Autodesk Inventor part; units mm, degrees
(part 2 of 2)
  circle A153 centre (-78.9982, -45.7929) radius 8 projected
  line L91 (-61.2813, 11.0455) -> (-50.1121, 17.3163) projected
  arc A154 (-102.4384, -34.1927) -> (-61.2813, 11.0455) centre (-111.1209, 15.0476) ccw projected
  line L92 (-102.4384, -34.1927) -> (-110.7406, -35.6566) projected
  line L93 (-110.7406, -35.6566) -> (-106.6609, -58.794) projected
  line L94 (-106.6609, -58.794) -> (-103.0049, -58.1494) projected
  arc A155 (-103.0049, -58.1494) -> (-82.3987, -72.578) centre (-78.9982, -45.7929) ccw projected
  line L95 (-82.3987, -72.578) -> (-81.7541, -76.234) projected
  line L96 (-81.7541, -76.234) -> (-73.8756, -74.8448) projected
  line L97 (-73.8756, -74.8448) -> (-28.2963, -90.7089) projected
  line L98 (-28.2963, -90.7089) -> (-30.7152, -97.3549) projected
  line L99 (-30.7152, -97.3549) -> (-15.0425, -100.6253) projected
  arc A156 (-15.0425, -100.6253) -> (-9.8606, -100.8097) centre (-10.3402, -41.375) ccw projected
  line L100 (-9.8606, -100.8097) -> (-9.8684, -99.8389) projected
  arc A157 (-7.953, -97.8245) -> (-9.8684, -99.8389) centre (-7.8685, -99.8228) ccw projected
  arc A158 (-7.953, -97.8245) -> (0.7138, -96.7831) centre (-10.3402, -41.375) ccw projected
  arc A159 (3.052, -98.2863) -> (0.7138, -96.7831) centre (1.1051, -98.7445) ccw projected
  line L101 (3.052, -98.2863) -> (3.358, -99.5868) projected
  arc A160 (3.358, -99.5868) -> (9.3677, -97.836) centre (-10.3402, -41.375) ccw projected
  line L102 (9.3677, -97.836) -> (20.2434, -92.7646) projected
  arc A161 (20.2434, -92.7646) -> (25.4476, -89.2862) centre (-10.3402, -41.375) ccw projected
  line L103 (25.4476, -89.2862) -> (24.6481, -88.2159) projected
  arc A162 (24.9994, -85.4585) -> (24.6481, -88.2159) centre (26.2504, -87.019) ccw projected
  arc A163 (24.9994, -85.4585) -> (31.3681, -79.4888) centre (-10.3402, -41.375) ccw projected
  arc A164 (34.1424, -79.3163) -> (31.3681, -79.4888) centre (32.8445, -80.838) ccw projected
  line L104 (34.1424, -79.3163) -> (34.8811, -79.9463) projected
  arc A165 (34.8811, -79.9463) -> (38.0707, -75.8583) centre (-10.3402, -41.375) ccw projected
  line L105 (38.0707, -75.8583) -> (45.6397, -61.75) projected
  line L106 (45.6397, -61.75) -> (38.9936, -59.3311) projected
  arc A166 (38.9936, -59.3311) -> (35.1261, -15.125) centre (-10.3402, -41.375) ccw projected
  line L107 (35.1261, -15.125) -> (41.2511, -11.5887) projected
  line L108 (41.2511, -11.5887) -> (31.3473, 0.9908) projected
  arc A167 (31.3473, 0.9908) -> (27.4962, 4.4629) centre (-10.3402, -41.375) ccw projected
  line L109 (27.4962, 4.4629) -> (26.8782, 3.7142) projected
  arc A168 (24.1161, 3.4024) -> (26.8782, 3.7142) centre (25.3358, 4.9874) ccw projected
  arc A169 (24.1161, 3.4024) -> (16.8075, 8.1755) centre (-10.3402, -41.375) ccw projected
  arc A170 (15.9827, 10.8299) -> (16.8075, 8.1755) centre (17.7685, 9.9295) ccw projected
  line L110 (15.9827, 10.8299) -> (16.5842, 12.0228) projected
  arc A171 (16.5842, 12.0228) -> (10.8551, 14.5447) centre (-10.3402, -41.375) ccw projected
  line L111 (10.8551, 14.5447) -> (-0.736, 17.6505) projected
  arc A172 (-0.736, 17.6505) -> (-6.9585, 18.3311) centre (-10.3402, -41.375) ccw projected
  line L112 (-6.9585, 18.3311) -> (-7.034, 16.9972) projected
  arc A173 (-9.0756, 15.1108) -> (-7.034, 16.9972) centre (-9.0308, 17.1103) ccw projected
  arc A174 (-9.0756, 15.1108) -> (-17.7916, 14.6315) centre (-10.3402, -41.375) ccw projected
  arc A175 (-20.0277, 16.2826) -> (-17.7916, 14.6315) centre (-18.0553, 16.614) ccw projected
  line L113 (-20.0277, 16.2826) -> (-20.1886, 17.24) projected
  arc A176 (-20.1886, 17.24) -> (-25.2597, 16.1586) centre (-10.3402, -41.375) ccw projected
  line L114 (-25.2597, 16.1586) -> (-40.1265, 10.2163) projected
  line L115 (-40.1265, 10.2163) -> (-50.1121, 17.3163) projected
  circle A177 centre (-103.9086, -54.247) radius 1.5 projected
  circle A178 centre (-13.7974, -97.2048) radius 1.5 projected
  circle A179 centre (20.8436, -88.2521) radius 1.5 projected
  circle A180 centre (28.1949, -0.8291) radius 1.5 projected
  circle A181 centre (-4.0964, 14.5795) radius 1.5 projected
  circle A182 centre (-23.4396, 13.0063) radius 1.5 projected
  circle A183 centre (12.2297, 10.2049) radius 1.5 projected
  circle A184 centre (34.6501, -74.6133) radius 1.5 projected
  circle A185 centre (5.5251, -95.3952) radius 1.5 projected
  circle A186 centre (-78.4226, -72.0925) radius 1.5 projected
  circle A187 centre (-10.3402, -41.375) radius 32.5 projected
  circle A188 centre (-78.9982, -45.7929) radius 12.5
  circle A189 centre (-78.9982, -45.7929) radius 21
  line L116 (-78.9982, -45.7929) -> (-99.6792, -49.4396)
  line L117 (-78.9982, -45.7929) -> (-86.1806, -65.5265)
  point P0 (0, 0)
  point P1 (-83.2735, -57.5391)
  point P2 (-91.3083, -47.9635)
  dimension "d58" = 25
  dimension "d59" = 42
  dimension "d60" = 60
  constraints: 4 end point, 2 centre point, 2 coincident, 2 point on circle, 1 parallel
  measures "d58" diameter of A188
  measures "d59" diameter of A189
  measures "d60" angle of L116 L117
extrude "Extrusion10" cut sketch "Sketch12" against normal blind 5 contours L116 A188 L117 A189
thicken "Thicken1" operation add thickness 1 both sides no extend neighbours yes toward (-0.6427876, -0.7660444, 0) faces at (-87.0331, -55.3685, 1.6667)
sketch "Sketch13" plane through (0, 0, 5) normal (0, 0, 1) x (1, 0, 0)
  line L0 (-83.6155, -58.4788) -> (-86.1806, -65.5265) projected
  arc A0 (-99.6792, -49.4396) -> (-86.1806, -65.5265) centre (-78.9982, -45.7929) ccw projected
  line L1 (-99.6792, -49.4396) -> (-92.2931, -48.1372) projected
  arc A1 (-92.2931, -48.1372) -> (-83.6155, -58.4788) centre (-78.9982, -45.7929) ccw projected
  arc A2 (-21.8035, -78.1288) -> (-9.3616, -79.8626) centre (-10.3402, -41.375) ccw projected
  line L2 (-9.3616, -79.8626) -> (-9.1582, -87.86) projected
  arc A3 (-24.6798, -85.6088) -> (-9.1582, -87.86) centre (-10.3402, -41.375) ccw projected
  line L3 (-24.6798, -85.6088) -> (-21.8314, -78.2051) projected
  arc A4 (-21.8314, -78.2051) -> (-21.8035, -78.1288) centre (-24.1646, -77.3074) ccw projected
  arc A5 (1.123, -4.6212) -> (-11.3188, -2.8874) centre (-10.3402, -41.375) ccw projected
  line L4 (-11.3188, -2.8874) -> (-11.6366, 9.6085) projected
  arc A6 (5.6174, 7.0642) -> (-11.6366, 9.6085) centre (-10.3402, -41.375) ccw projected
  line L5 (5.6174, 7.0642) -> (1.1509, -4.5449) projected
  arc A7 (1.1509, -4.5449) -> (1.123, -4.6212) centre (3.4842, -5.4426) ccw projected
  arc A8 (4.1075, -90.2858) -> (19.7424, -82.5579) centre (-10.3402, -41.375) ccw projected
  line L6 (4.1075, -90.2858) -> (0.5664, -78.2978) projected
  arc A9 (0.5664, -78.2978) -> (11.8719, -72.8214) centre (-10.3402, -41.375) ccw projected
  arc A10 (11.8719, -72.8214) -> (11.9219, -72.8853) centre (13.8659, -71.3135) ccw projected
  line L7 (11.9219, -72.8853) -> (19.7424, -82.5579) projected
  arc A11 (-59.922, -29.4317) -> (-61.047, -46.8359) centre (-10.3402, -41.375) ccw projected
  line L8 (-59.922, -29.4317) -> (-47.7696, -32.359) projected
  arc A12 (-47.7696, -32.359) -> (-48.6796, -44.888) centre (-10.3402, -41.375) ccw projected
  arc A13 (-48.6796, -44.888) -> (-48.76, -44.8994) centre (-48.3708, -47.3689) ccw projected
  line L9 (-48.76, -44.8994) -> (-61.047, -46.8359) projected
  arc A14 (-36.4384, -13.0706) -> (-44.1607, -22.9787) centre (-10.3402, -41.375) ccw projected
  line L10 (-44.1607, -22.9787) -> (-55.1414, -17.0059) projected
  arc A15 (-44.311, -3.3357) -> (-55.1414, -17.0059) centre (-10.3402, -41.375) ccw projected
  line L11 (-44.311, -3.3357) -> (-36.4904, -13.0083) projected
  arc A16 (-36.4904, -13.0083) -> (-36.4384, -13.0706) centre (-34.5464, -11.4365) ccw projected
  arc A17 (34.8667, -52.2645) -> (35.9156, -36.6156) centre (-10.3402, -41.375) ccw projected
  line L12 (34.8667, -52.2645) -> (27.0892, -50.391) projected
  arc A18 (27.0892, -50.391) -> (27.9992, -37.862) centre (-10.3402, -41.375) ccw projected
  arc A19 (27.9992, -37.862) -> (28.0796, -37.8506) centre (27.6903, -35.3811) ccw projected
  line L13 (28.0796, -37.8506) -> (35.9156, -36.6156) projected
  arc A20 (-26.4675, -76.3344) -> (-26.4979, -76.4097) centre (-24.1646, -77.3074) ccw projected
  line L14 (-26.4979, -76.4097) -> (-29.3464, -83.8134) projected
  arc A21 (-42.3743, -75.0806) -> (-29.3464, -83.8134) centre (-10.3402, -41.375) ccw projected
  line L15 (-42.3743, -75.0806) -> (-36.863, -69.2818) projected
  arc A22 (-36.863, -69.2818) -> (-26.4675, -76.3344) centre (-10.3402, -41.375) ccw projected
  arc A23 (5.7871, -6.4156) -> (5.8175, -6.3403) centre (3.4842, -5.4426) ccw projected
  line L16 (5.8175, -6.3403) -> (10.2839, 5.2688) projected
  arc A24 (24.7939, -4.4075) -> (10.2839, 5.2688) centre (-10.3402, -41.375) ccw projected
  line L17 (24.7939, -4.4075) -> (16.1826, -13.4682) projected
  arc A25 (16.1826, -13.4682) -> (5.7871, -6.4156) centre (-10.3402, -41.375) ccw projected
  line L18 (23.6306, -79.4143) -> (15.81, -69.7417) projected
  arc A26 (15.81, -69.7417) -> (15.7579, -69.6794) centre (13.8659, -71.3135) ccw projected
  arc A27 (15.7579, -69.6794) -> (23.4803, -59.7713) centre (-10.3402, -41.375) ccw projected
  line L19 (23.4803, -59.7713) -> (34.461, -65.7441) projected
  arc A28 (23.6306, -79.4143) -> (34.461, -65.7441) centre (-10.3402, -41.375) ccw projected
  line L20 (-60.2686, -51.7749) -> (-47.9816, -49.8384) projected
  arc A29 (-47.9816, -49.8384) -> (-47.9016, -49.8245) centre (-48.3708, -47.3689) ccw projected
  arc A30 (-47.9016, -49.8245) -> (-43.1821, -61.4663) centre (-10.3402, -41.375) ccw projected
  line L21 (-43.1821, -61.4663) -> (-53.8451, -67.9894) projected
  arc A31 (-60.2686, -51.7749) -> (-53.8451, -67.9894) centre (-10.3402, -41.375) ccw projected
  arc A32 (-32.5523, -9.9286) -> (-32.6023, -9.8647) centre (-34.5464, -11.4365) ccw projected
  line L22 (-32.6023, -9.8647) -> (-40.4229, -0.1921) projected
  arc A33 (-24.7879, 7.5358) -> (-40.4229, -0.1921) centre (-10.3402, -41.375) ccw projected
  line L23 (-24.7879, 7.5358) -> (-21.2468, -4.4522) projected
  arc A34 (-21.2468, -4.4522) -> (-32.5523, -9.9286) centre (-10.3402, -41.375) ccw projected
  line L24 (35.1371, -31.6766) -> (27.3011, -32.9116) projected
  arc A35 (27.3011, -32.9116) -> (27.2212, -32.9255) centre (27.6903, -35.3811) ccw projected
  arc A36 (27.2212, -32.9255) -> (22.5017, -21.2837) centre (-10.3402, -41.375) ccw projected
  line L25 (22.5017, -21.2837) -> (29.326, -17.1089) projected
  arc A37 (35.1371, -31.6766) -> (29.326, -17.1089) centre (-10.3402, -41.375) ccw projected
  circle A38 centre (-81.1726, -30.4864) radius 2.1 projected
  circle A39 centre (-65.5868, -14.9006) radius 2.1 projected
  circle A40 centre (-101.657, -38.6244) radius 2.1 projected
  circle A41 centre (-57.4488, 5.5838) radius 2.1 projected
  circle A42 centre (-78.9982, -45.7929) radius 8 projected
  line L26 (-61.2813, 11.0455) -> (-50.1121, 17.3163) projected
  arc A43 (-102.4384, -34.1927) -> (-61.2813, 11.0455) centre (-111.1209, 15.0476) ccw projected
  line L27 (-102.4384, -34.1927) -> (-110.7406, -35.6566) projected
  line L28 (-110.7406, -35.6566) -> (-106.6609, -58.794) projected
  line L29 (-106.6609, -58.794) -> (-103.0049, -58.1494) projected
  arc A44 (-103.0049, -58.1494) -> (-82.3987, -72.578) centre (-78.9982, -45.7929) ccw projected
  line L30 (-82.3987, -72.578) -> (-81.7541, -76.234) projected
  line L31 (-81.7541, -76.234) -> (-73.8756, -74.8448) projected
  line L32 (-73.8756, -74.8448) -> (-28.2963, -90.7089) projected
  line L33 (-28.2963, -90.7089) -> (-30.7152, -97.3549) projected
  line L34 (-30.7152, -97.3549) -> (-15.0425, -100.6253) projected
  arc A45 (-15.0425, -100.6253) -> (-9.8606, -100.8097) centre (-10.3402, -41.375) ccw projected
  line L35 (-9.8606, -100.8097) -> (-9.8684, -99.8389) projected
  arc A46 (-7.953, -97.8245) -> (-9.8684, -99.8389) centre (-7.8685, -99.8228) ccw projected
  arc A47 (-7.953, -97.8245) -> (0.7138, -96.7831) centre (-10.3402, -41.375) ccw projected
  arc A48 (3.052, -98.2863) -> (0.7138, -96.7831) centre (1.1051, -98.7445) ccw projected
  line L36 (3.052, -98.2863) -> (3.358, -99.5868) projected
  arc A49 (3.358, -99.5868) -> (9.3677, -97.836) centre (-10.3402, -41.375) ccw projected
  line L37 (9.3677, -97.836) -> (20.2434, -92.7646) projected
  arc A50 (20.2434, -92.7646) -> (25.4476, -89.2862) centre (-10.3402, -41.375) ccw projected
  line L38 (25.4476, -89.2862) -> (24.6481, -88.2159) projected
  arc A51 (24.9994, -85.4585) -> (24.6481, -88.2159) centre (26.2504, -87.019) ccw projected
  arc A52 (24.9994, -85.4585) -> (31.3681, -79.4888) centre (-10.3402, -41.375) ccw projected
  arc A53 (34.1424, -79.3163) -> (31.3681, -79.4888) centre (32.8445, -80.838) ccw projected
  line L39 (34.1424, -79.3163) -> (34.8811, -79.9463) projected
  arc A54 (34.8811, -79.9463) -> (38.0707, -75.8583) centre (-10.3402, -41.375) ccw projected
  line L40 (38.0707, -75.8583) -> (45.6397, -61.75) projected
  line L41 (45.6397, -61.75) -> (38.9936, -59.3311) projected
  arc A55 (38.9936, -59.3311) -> (35.1261, -15.125) centre (-10.3402, -41.375) ccw projected
  line L42 (35.1261, -15.125) -> (41.2511, -11.5887) projected
  line L43 (41.2511, -11.5887) -> (31.3473, 0.9908) projected
  arc A56 (31.3473, 0.9908) -> (27.4962, 4.4629) centre (-10.3402, -41.375) ccw projected
  line L44 (27.4962, 4.4629) -> (26.8782, 3.7142) projected
  arc A57 (24.1161, 3.4024) -> (26.8782, 3.7142) centre (25.3358, 4.9874) ccw projected
  arc A58 (24.1161, 3.4024) -> (16.8075, 8.1755) centre (-10.3402, -41.375) ccw projected
  arc A59 (15.9827, 10.8299) -> (16.8075, 8.1755) centre (17.7685, 9.9295) ccw projected
  line L45 (15.9827, 10.8299) -> (16.5842, 12.0228) projected
  arc A60 (16.5842, 12.0228) -> (10.8551, 14.5447) centre (-10.3402, -41.375) ccw projected
  line L46 (10.8551, 14.5447) -> (-0.736, 17.6505) projected
  arc A61 (-0.736, 17.6505) -> (-6.9585, 18.3311) centre (-10.3402, -41.375) ccw projected
  line L47 (-6.9585, 18.3311) -> (-7.034, 16.9972) projected
  arc A62 (-9.0756, 15.1108) -> (-7.034, 16.9972) centre (-9.0308, 17.1103) ccw projected
  arc A63 (-9.0756, 15.1108) -> (-17.7916, 14.6315) centre (-10.3402, -41.375) ccw projected
  arc A64 (-20.0277, 16.2826) -> (-17.7916, 14.6315) centre (-18.0553, 16.614) ccw projected
  line L48 (-20.0277, 16.2826) -> (-20.1886, 17.24) projected
  arc A65 (-20.1886, 17.24) -> (-25.2597, 16.1586) centre (-10.3402, -41.375) ccw projected
  line L49 (-25.2597, 16.1586) -> (-40.1265, 10.2163) projected
  line L50 (-40.1265, 10.2163) -> (-50.1121, 17.3163) projected
  circle A66 centre (-103.9086, -54.247) radius 1.5 projected
  circle A67 centre (-13.7974, -97.2048) radius 1.5 projected
  circle A68 centre (20.8436, -88.2521) radius 1.5 projected
  circle A69 centre (28.1949, -0.8291) radius 1.5 projected
  circle A70 centre (-4.0964, 14.5795) radius 1.5 projected
  circle A71 centre (-23.4396, 13.0063) radius 1.5 projected
  circle A72 centre (12.2297, 10.2049) radius 1.5 projected
  circle A73 centre (34.6501, -74.6133) radius 1.5 projected
  circle A74 centre (5.5251, -95.3952) radius 1.5 projected
  circle A75 centre (-78.4226, -72.0925) radius 1.5 projected
  circle A76 centre (-10.3402, -41.375) radius 32.5 projected
  circle A77 centre (-78.9982, -45.7929) radius 13.5
  circle A78 centre (-10.3402, -41.375) radius 57.5
  line L51 (-79.8686, -59.2649) -> (-56.0684, -76.2345)
  point P0 (0, 0)
  point P1 (-66.893, -51.769)
  dimension "d65" = 27
  dimension "d66" = 115
  constraints: 2 coincident, 2 end point, 6 other
extrude "Extrusion11" cut sketch "Sketch13" against normal blind 5 contours A77 A78 L51
fillet "Fillet1" radius 2 3 edges at (-79.8686, -59.2649, 2.5) (-66.893, -51.769, 2.5) (-56.0684, -76.2345, 2.5)
fillet "Fillet2" radius 2 4 edges at (-83.6155, -58.4788, 2.5) (-92.2931, -48.1372, 2.5) (-99.6792, -49.4396, 2.5) (-86.1806, -65.5265, 2.5)
sketch "Sketch14" plane through (0, 0, 5) normal (0, 0, 1) x (1, 0, 0)
  arc A0 (-75.0894, -58.7147) -> (-69.3018, -55.186) centre (-78.9982, -45.7929) ccw projected
  arc A1 (-65.9317, -56.0665) -> (-69.3018, -55.186) centre (-67.8653, -56.5775) ccw projected
  arc A2 (-65.9317, -56.0665) -> (-61.4204, -67.7771) centre (-10.3402, -41.375) ccw projected
  arc A3 (-64.3581, -70.3239) -> (-61.4204, -67.7771) centre (-63.1971, -68.6954) ccw projected
  line L0 (-64.3581, -70.3239) -> (-75.6714, -62.2575) projected
  arc A4 (-75.0894, -58.7147) -> (-75.6714, -62.2575) centre (-74.5103, -60.629) ccw projected
  line L1 (-84.2552, -60.2364) -> (-85.4605, -63.5479) projected
  arc A5 (-88.218, -64.6608) -> (-85.4605, -63.5479) centre (-87.3399, -62.8639) ccw projected
  arc A6 (-99.1804, -51.5962) -> (-88.218, -64.6608) centre (-78.9982, -45.7929) ccw projected
  arc A7 (-97.6056, -49.0739) -> (-99.1804, -51.5962) centre (-97.2583, -51.0435) ccw projected
  line L2 (-97.6056, -49.0739) -> (-94.1351, -48.462) projected
  arc A8 (-91.8795, -49.8331) -> (-94.1351, -48.462) centre (-93.7878, -50.4316) ccw projected
  arc A9 (-91.8795, -49.8331) -> (-85.2138, -57.777) centre (-78.9982, -45.7929) ccw projected
  arc A10 (-84.2552, -60.2364) -> (-85.2138, -57.777) centre (-86.1346, -59.5524) ccw projected
  arc A11 (-21.8035, -78.1288) -> (-9.3616, -79.8626) centre (-10.3402, -41.375) ccw projected
  line L3 (-9.3616, -79.8626) -> (-9.1582, -87.86) projected
  arc A12 (-24.6798, -85.6088) -> (-9.1582, -87.86) centre (-10.3402, -41.375) ccw projected
  line L4 (-24.6798, -85.6088) -> (-21.8314, -78.2051) projected
  arc A13 (-21.8314, -78.2051) -> (-21.8035, -78.1288) centre (-24.1646, -77.3074) ccw projected
  arc A14 (1.123, -4.6212) -> (-11.3188, -2.8874) centre (-10.3402, -41.375) ccw projected
  line L5 (-11.3188, -2.8874) -> (-11.6366, 9.6085) projected
  arc A15 (5.6174, 7.0642) -> (-11.6366, 9.6085) centre (-10.3402, -41.375) ccw projected
  line L6 (5.6174, 7.0642) -> (1.1509, -4.5449) projected
  arc A16 (1.1509, -4.5449) -> (1.123, -4.6212) centre (3.4842, -5.4426) ccw projected
  arc A17 (4.1075, -90.2858) -> (19.7424, -82.5579) centre (-10.3402, -41.375) ccw projected
  line L7 (4.1075, -90.2858) -> (0.5664, -78.2978) projected
  arc A18 (0.5664, -78.2978) -> (11.8719, -72.8214) centre (-10.3402, -41.375) ccw projected
  arc A19 (11.8719, -72.8214) -> (11.9219, -72.8853) centre (13.8659, -71.3135) ccw projected
  line L8 (11.9219, -72.8853) -> (19.7424, -82.5579) projected
  arc A20 (-59.922, -29.4317) -> (-61.047, -46.8359) centre (-10.3402, -41.375) ccw projected
  line L9 (-59.922, -29.4317) -> (-47.7696, -32.359) projected
  arc A21 (-47.7696, -32.359) -> (-48.6796, -44.888) centre (-10.3402, -41.375) ccw projected
  arc A22 (-48.6796, -44.888) -> (-48.76, -44.8994) centre (-48.3708, -47.3689) ccw projected
  line L10 (-48.76, -44.8994) -> (-61.047, -46.8359) projected
  arc A23 (-36.4384, -13.0706) -> (-44.1607, -22.9787) centre (-10.3402, -41.375) ccw projected
  line L11 (-44.1607, -22.9787) -> (-55.1414, -17.0059) projected
  arc A24 (-44.311, -3.3357) -> (-55.1414, -17.0059) centre (-10.3402, -41.375) ccw projected
  line L12 (-44.311, -3.3357) -> (-36.4904, -13.0083) projected
  arc A25 (-36.4904, -13.0083) -> (-36.4384, -13.0706) centre (-34.5464, -11.4365) ccw projected
  arc A26 (34.8667, -52.2645) -> (35.9156, -36.6156) centre (-10.3402, -41.375) ccw projected
  line L13 (34.8667, -52.2645) -> (27.0892, -50.391) projected
  arc A27 (27.0892, -50.391) -> (27.9992, -37.862) centre (-10.3402, -41.375) ccw projected
  arc A28 (27.9992, -37.862) -> (28.0796, -37.8506) centre (27.6903, -35.3811) ccw projected
  line L14 (28.0796, -37.8506) -> (35.9156, -36.6156) projected
  arc A29 (-26.4675, -76.3344) -> (-26.4979, -76.4097) centre (-24.1646, -77.3074) ccw projected
  line L15 (-26.4979, -76.4097) -> (-29.3464, -83.8134) projected
  arc A30 (-42.3743, -75.0806) -> (-29.3464, -83.8134) centre (-10.3402, -41.375) ccw projected
  line L16 (-42.3743, -75.0806) -> (-36.863, -69.2818) projected
  arc A31 (-36.863, -69.2818) -> (-26.4675, -76.3344) centre (-10.3402, -41.375) ccw projected
  arc A32 (5.7871, -6.4156) -> (5.8175, -6.3403) centre (3.4842, -5.4426) ccw projected
  line L17 (5.8175, -6.3403) -> (10.2839, 5.2688) projected
  arc A33 (24.7939, -4.4075) -> (10.2839, 5.2688) centre (-10.3402, -41.375) ccw projected
  line L18 (24.7939, -4.4075) -> (16.1826, -13.4682) projected
  arc A34 (16.1826, -13.4682) -> (5.7871, -6.4156) centre (-10.3402, -41.375) ccw projected
  line L19 (23.6306, -79.4143) -> (15.81, -69.7417) projected
  arc A35 (15.81, -69.7417) -> (15.7579, -69.6794) centre (13.8659, -71.3135) ccw projected
  arc A36 (15.7579, -69.6794) -> (23.4803, -59.7713) centre (-10.3402, -41.375) ccw projected
  line L20 (23.4803, -59.7713) -> (34.461, -65.7441) projected
  arc A37 (23.6306, -79.4143) -> (34.461, -65.7441) centre (-10.3402, -41.375) ccw projected
  line L21 (-60.2686, -51.7749) -> (-47.9816, -49.8384) projected
  arc A38 (-47.9816, -49.8384) -> (-47.9016, -49.8245) centre (-48.3708, -47.3689) ccw projected
  arc A39 (-47.9016, -49.8245) -> (-43.1821, -61.4663) centre (-10.3402, -41.375) ccw projected
  line L22 (-43.1821, -61.4663) -> (-53.8451, -67.9894) projected
  arc A40 (-60.2686, -51.7749) -> (-53.8451, -67.9894) centre (-10.3402, -41.375) ccw projected
  arc A41 (-32.5523, -9.9286) -> (-32.6023, -9.8647) centre (-34.5464, -11.4365) ccw projected
  line L23 (-32.6023, -9.8647) -> (-40.4229, -0.1921) projected
  arc A42 (-24.7879, 7.5358) -> (-40.4229, -0.1921) centre (-10.3402, -41.375) ccw projected
  line L24 (-24.7879, 7.5358) -> (-21.2468, -4.4522) projected
  arc A43 (-21.2468, -4.4522) -> (-32.5523, -9.9286) centre (-10.3402, -41.375) ccw projected
  line L25 (35.1371, -31.6766) -> (27.3011, -32.9116) projected
  arc A44 (27.3011, -32.9116) -> (27.2212, -32.9255) centre (27.6903, -35.3811) ccw projected
  arc A45 (27.2212, -32.9255) -> (22.5017, -21.2837) centre (-10.3402, -41.375) ccw projected
  line L26 (22.5017, -21.2837) -> (29.326, -17.1089) projected
  arc A46 (35.1371, -31.6766) -> (29.326, -17.1089) centre (-10.3402, -41.375) ccw projected
  circle A47 centre (-81.1726, -30.4864) radius 2.1 projected
  circle A48 centre (-65.5868, -14.9006) radius 2.1 projected
  circle A49 centre (-101.657, -38.6244) radius 2.1 projected
  circle A50 centre (-57.4488, 5.5838) radius 2.1 projected
  circle A51 centre (-78.9982, -45.7929) radius 8 projected
  line L27 (-61.2813, 11.0455) -> (-50.1121, 17.3163) projected
  arc A52 (-102.4384, -34.1927) -> (-61.2813, 11.0455) centre (-111.1209, 15.0476) ccw projected
  line L28 (-102.4384, -34.1927) -> (-110.7406, -35.6566) projected
  line L29 (-110.7406, -35.6566) -> (-106.6609, -58.794) projected
  line L30 (-106.6609, -58.794) -> (-103.0049, -58.1494) projected
  arc A53 (-103.0049, -58.1494) -> (-82.3987, -72.578) centre (-78.9982, -45.7929) ccw projected
  line L31 (-82.3987, -72.578) -> (-81.7541, -76.234) projected
  line L32 (-81.7541, -76.234) -> (-73.8756, -74.8448) projected
  line L33 (-73.8756, -74.8448) -> (-28.2963, -90.7089) projected
  line L34 (-28.2963, -90.7089) -> (-30.7152, -97.3549) projected
  line L35 (-30.7152, -97.3549) -> (-15.0425, -100.6253) projected
  arc A54 (-15.0425, -100.6253) -> (-9.8606, -100.8097) centre (-10.3402, -41.375) ccw projected
  line L36 (-9.8606, -100.8097) -> (-9.8684, -99.8389) projected
  arc A55 (-7.953, -97.8245) -> (-9.8684, -99.8389) centre (-7.8685, -99.8228) ccw projected
  arc A56 (-7.953, -97.8245) -> (0.7138, -96.7831) centre (-10.3402, -41.375) ccw projected
  arc A57 (3.052, -98.2863) -> (0.7138, -96.7831) centre (1.1051, -98.7445) ccw projected
  line L37 (3.052, -98.2863) -> (3.358, -99.5868) projected
  arc A58 (3.358, -99.5868) -> (9.3677, -97.836) centre (-10.3402, -41.375) ccw projected
  line L38 (9.3677, -97.836) -> (20.2434, -92.7646) projected
  arc A59 (20.2434, -92.7646) -> (25.4476, -89.2862) centre (-10.3402, -41.375) ccw projected
  line L39 (25.4476, -89.2862) -> (24.6481, -88.2159) projected
  arc A60 (24.9994, -85.4585) -> (24.6481, -88.2159) centre (26.2504, -87.019) ccw projected
  arc A61 (24.9994, -85.4585) -> (31.3681, -79.4888) centre (-10.3402, -41.375) ccw projected
  arc A62 (34.1424, -79.3163) -> (31.3681, -79.4888) centre (32.8445, -80.838) ccw projected
  line L40 (34.1424, -79.3163) -> (34.8811, -79.9463) projected
  arc A63 (34.8811, -79.9463) -> (38.0707, -75.8583) centre (-10.3402, -41.375) ccw projected
  line L41 (38.0707, -75.8583) -> (45.6397, -61.75) projected
  line L42 (45.6397, -61.75) -> (38.9936, -59.3311) projected
  arc A64 (38.9936, -59.3311) -> (35.1261, -15.125) centre (-10.3402, -41.375) ccw projected
  line L43 (35.1261, -15.125) -> (41.2511, -11.5887) projected
  line L44 (41.2511, -11.5887) -> (31.3473, 0.9908) projected
  arc A65 (31.3473, 0.9908) -> (27.4962, 4.4629) centre (-10.3402, -41.375) ccw projected
  line L45 (27.4962, 4.4629) -> (26.8782, 3.7142) projected
  arc A66 (24.1161, 3.4024) -> (26.8782, 3.7142) centre (25.3358, 4.9874) ccw projected
  arc A67 (24.1161, 3.4024) -> (16.8075, 8.1755) centre (-10.3402, -41.375) ccw projected
  arc A68 (15.9827, 10.8299) -> (16.8075, 8.1755) centre (17.7685, 9.9295) ccw projected
  line L46 (15.9827, 10.8299) -> (16.5842, 12.0228) projected
  arc A69 (16.5842, 12.0228) -> (10.8551, 14.5447) centre (-10.3402, -41.375) ccw projected
  line L47 (10.8551, 14.5447) -> (-0.736, 17.6505) projected
  arc A70 (-0.736, 17.6505) -> (-6.9585, 18.3311) centre (-10.3402, -41.375) ccw projected
  line L48 (-6.9585, 18.3311) -> (-7.034, 16.9972) projected
  arc A71 (-9.0756, 15.1108) -> (-7.034, 16.9972) centre (-9.0308, 17.1103) ccw projected
  arc A72 (-9.0756, 15.1108) -> (-17.7916, 14.6315) centre (-10.3402, -41.375) ccw projected
  arc A73 (-20.0277, 16.2826) -> (-17.7916, 14.6315) centre (-18.0553, 16.614) ccw projected
  line L49 (-20.0277, 16.2826) -> (-20.1886, 17.24) projected
  arc A74 (-20.1886, 17.24) -> (-25.2597, 16.1586) centre (-10.3402, -41.375) ccw projected
  line L50 (-25.2597, 16.1586) -> (-40.1265, 10.2163) projected
  line L51 (-40.1265, 10.2163) -> (-50.1121, 17.3163) projected
  circle A75 centre (-103.9086, -54.247) radius 1.5 projected
  circle A76 centre (-13.7974, -97.2048) radius 1.5 projected
  circle A77 centre (20.8436, -88.2521) radius 1.5 projected
  circle A78 centre (28.1949, -0.8291) radius 1.5 projected
  circle A79 centre (-4.0964, 14.5795) radius 1.5 projected
  circle A80 centre (-23.4396, 13.0063) radius 1.5 projected
  circle A81 centre (12.2297, 10.2049) radius 1.5 projected
  circle A82 centre (34.6501, -74.6133) radius 1.5 projected
  circle A83 centre (5.5251, -95.3952) radius 1.5 projected
  circle A84 centre (-78.4226, -72.0925) radius 1.5 projected
  circle A85 centre (-10.3402, -41.375) radius 32.5 projected
  circle A86 centre (-78.9982, -45.7929) radius 13.5
  circle A87 centre (-111.1209, 15.0476) radius 58.5
  circle A88 centre (-10.3402, -41.375) radius 57
  point P0 (0, 0)
  point P1 (-67.2934, -39.0663)
  point P2 (-60.0763, -13.5305)
  point P3 (-76.9663, -32.4467)
  dimension "d71" = 27
  dimension "d72" = 117
  dimension "d73" = 114
  constraints: 3 centre point, 3 coincident
  measures "d71" diameter of A86
  measures "d72" diameter of A87
  measures "d73" diameter of A88
extrude "Extrusion12" cut sketch "Sketch14" against normal blind 5 contours A86 A87 A88
fillet "Fillet3" radius 2 3 edges at (-60.0763, -13.5305, 2.5) (-76.9663, -32.4467, 2.5) (-67.2934, -39.0663, 2.5)
fillet "Fillet4" radius 3 24 edges at (-60.2686, -51.7749, 2.5) (-53.8451, -67.9894, 2.5) (-61.047, -46.8359, 2.5) (-59.922, -29.4317, 2.5) (-55.1414, -17.0059, 2.5) (-44.311, -3.3357, 2.5) (-24.7879, 7.5358, 2.5) (-40.4229, -0.1921, 2.5) (-11.6366, 9.6085, 2.5) (5.6174, 7.0642, 2.5) (10.2839, 5.2688, 2.5) (24.7939, -4.4075, 2.5) (29.326, -17.1089, 2.5) (35.1371, -31.6766, 2.5) (35.9156, -36.6156, 2.5) (34.8667, -52.2645, 2.5) (34.461, -65.7441, 2.5) (23.6306, -79.4143, 2.5) (19.7424, -82.5579, 2.5) (4.1075, -90.2858, 2.5) (-9.1582, -87.86, 2.5) (-24.6798, -85.6088, 2.5) (-29.3464, -83.8134, 2.5) (-42.3743, -75.0806, 2.5)
fillet "Fillet5" radius 3 24 edges at (-43.1821, -61.4663, 2.5) (-47.9016, -49.8245, 2.5) (-48.6796, -44.888, 2.5) (-47.7696, -32.359, 2.5) (-44.1607, -22.9787, 2.5) (-36.4384, -13.0706, 2.5) (-32.5523, -9.9286, 2.5) (-21.2468, -4.4522, 2.5) (-11.3188, -2.8874, 2.5) (1.123, -4.6212, 2.5) (5.7871, -6.4156, 2.5) (16.1826, -13.4682, 2.5) (22.5017, -21.2837, 2.5) (27.9992, -37.862, 2.5) (27.2212, -32.9255, 2.5) (27.0892, -50.391, 2.5) (23.4803, -59.7713, 2.5) (11.8719, -72.8214, 2.5) (15.7579, -69.6794, 2.5) (0.5664, -78.2978, 2.5) (-9.3616, -79.8626, 2.5) (-26.4675, -76.3344, 2.5) (-21.8035, -78.1288, 2.5) (-36.863, -69.2818, 2.5)
sketch "Sketch15" plane through (0, 0, 5) normal (0, 0, 1) x (1, 0, 0)
  arc A0 (-70.1886, -35.5635) -> (-73.474, -33.4749) centre (-78.9982, -45.7929) ccw projected
  arc A1 (-73.9272, -30.1063) -> (-73.474, -33.4749) centre (-72.6556, -31.6501) ccw projected
  arc A2 (-73.9272, -30.1063) -> (-68.9821, -25.5304) centre (-111.1209, 15.0476) ccw projected
  arc A3 (-65.6025, -27.4078) -> (-68.9821, -25.5304) centre (-67.5415, -26.9177) ccw projected
  arc A4 (-65.6025, -27.4078) -> (-66.899, -34.2964) centre (-10.3402, -41.375) ccw projected
  arc A5 (-70.1886, -35.5635) -> (-66.899, -34.2964) centre (-68.8835, -34.0481) ccw projected
  arc A6 (-75.0894, -58.7147) -> (-69.3018, -55.186) centre (-78.9982, -45.7929) ccw projected
  arc A7 (-65.9317, -56.0665) -> (-69.3018, -55.186) centre (-67.8653, -56.5775) ccw projected
  arc A8 (-65.9317, -56.0665) -> (-61.4204, -67.7771) centre (-10.3402, -41.375) ccw projected
  arc A9 (-64.3581, -70.3239) -> (-61.4204, -67.7771) centre (-63.1971, -68.6954) ccw projected
  line L0 (-64.3581, -70.3239) -> (-75.6714, -62.2575) projected
  arc A10 (-75.0894, -58.7147) -> (-75.6714, -62.2575) centre (-74.5103, -60.629) ccw projected
  line L1 (-84.2552, -60.2364) -> (-85.4605, -63.5479) projected
  arc A11 (-88.218, -64.6608) -> (-85.4605, -63.5479) centre (-87.3399, -62.8639) ccw projected
  arc A12 (-99.1804, -51.5962) -> (-88.218, -64.6608) centre (-78.9982, -45.7929) ccw projected
  arc A13 (-97.6056, -49.0739) -> (-99.1804, -51.5962) centre (-97.2583, -51.0435) ccw projected
  line L2 (-97.6056, -49.0739) -> (-94.1351, -48.462) projected
  arc A14 (-91.8795, -49.8331) -> (-94.1351, -48.462) centre (-93.7878, -50.4316) ccw projected
  arc A15 (-91.8795, -49.8331) -> (-85.2138, -57.777) centre (-78.9982, -45.7929) ccw projected
  arc A16 (-84.2552, -60.2364) -> (-85.2138, -57.777) centre (-86.1346, -59.5524) ccw projected
  arc A17 (-19.2806, -78.8226) -> (-12.1464, -79.8326) centre (-10.3402, -41.375) ccw projected
  arc A18 (-9.2881, -82.7531) -> (-12.1464, -79.8326) centre (-12.2871, -82.8293) ccw projected
  line L3 (-9.2881, -82.7531) -> (-9.2371, -84.7574) projected
  arc A19 (-12.3669, -87.8308) -> (-9.2371, -84.7574) centre (-12.2362, -84.8337) ccw projected
  arc A20 (-21.416, -86.5367) -> (-12.3669, -87.8308) centre (-10.3402, -41.375) ccw projected
  arc A21 (-23.5014, -82.5458) -> (-21.416, -86.5367) centre (-20.7015, -83.623) ccw projected
  line L4 (-23.5014, -82.5458) -> (-22.7771, -80.6633) projected
  arc A22 (-19.2806, -78.8226) -> (-22.7771, -80.6633) centre (-19.9772, -81.7406) ccw projected
  arc A23 (-1.3999, -3.9274) -> (-8.534, -2.9174) centre (-10.3402, -41.375) ccw projected
  arc A24 (-11.3923, 0.0031) -> (-8.534, -2.9174) centre (-8.3933, 0.0793) ccw projected
  line L5 (-11.3923, 0.0031) -> (-11.5579, 6.5157) projected
  arc A25 (-8.4476, 9.5899) -> (-11.5579, 6.5157) centre (-8.5589, 6.5919) ccw projected
  arc A26 (2.398, 8.0086) -> (-8.4476, 9.5899) centre (-10.3402, -41.375) ccw projected
  arc A27 (4.4486, 4.0264) -> (2.398, 8.0086) centre (1.6487, 5.1037) ccw projected
  line L6 (4.4486, 4.0264) -> (2.0967, -2.0867) projected
  arc A28 (-1.3999, -3.9274) -> (2.0967, -2.0867) centre (-0.7032, -1.0094) ccw projected
  arc A29 (7.1362, -89.2872) -> (16.9696, -84.4467) centre (-10.3402, -41.375) ccw projected
  arc A30 (3.231, -87.3187) -> (7.1362, -89.2872) centre (6.1081, -86.4688) ccw projected
  line L7 (3.231, -87.3187) -> (1.3855, -81.0708) projected
  arc A31 (3.207, -77.4128) -> (1.3855, -81.0708) centre (4.2626, -80.221) ccw projected
  arc A32 (3.207, -77.4128) -> (9.6846, -74.2574) centre (-10.3402, -41.375) ccw projected
  arc A33 (13.5779, -74.9335) -> (9.6846, -74.2574) centre (11.245, -76.8197) ccw projected
  line L8 (13.5779, -74.9335) -> (17.696, -80.0269) projected
  arc A34 (16.9696, -84.4467) -> (17.696, -80.0269) centre (15.3632, -81.9131) ccw projected
  arc A35 (-60.5716, -32.5539) -> (-61.2963, -43.4902) centre (-10.3402, -41.375) ccw projected
  arc A36 (-56.9142, -30.1562) -> (-60.5716, -32.5539) centre (-57.6168, -33.0728) ccw projected
  line L9 (-56.9142, -30.1562) -> (-50.5807, -31.6818) projected
  arc A37 (-48.3235, -35.0883) -> (-50.5807, -31.6818) centre (-51.2832, -34.5984) ccw projected
  arc A38 (-48.3235, -35.0883) -> (-48.8297, -42.2758) centre (-10.3402, -41.375) ccw projected
  arc A39 (-51.3618, -45.3094) -> (-48.8297, -42.2758) centre (-51.8289, -42.346) ccw projected
  line L10 (-51.3618, -45.3094) -> (-57.8319, -46.3292) projected
  arc A40 (-61.2963, -43.4902) -> (-57.8319, -46.3292) centre (-58.2989, -43.3657) ccw projected
  arc A41 (-38.3006, -14.9086) -> (-42.7424, -20.582) centre (-10.3402, -41.375) ccw projected
  arc A42 (-46.7007, -21.5971) -> (-42.7424, -20.582) centre (-45.2672, -18.9618) ccw projected
  line L11 (-46.7007, -21.5971) -> (-52.4236, -18.4842) projected
  arc A43 (-53.5308, -14.2535) -> (-52.4236, -18.4842) centre (-50.9901, -15.8489) ccw projected
  arc A44 (-46.7385, -5.6516) -> (-53.5308, -14.2535) centre (-10.3402, -41.375) ccw projected
  arc A45 (-42.2646, -5.8668) -> (-46.7385, -5.6516) centre (-44.5975, -7.753) ccw projected
  line L12 (-42.2646, -5.8668) -> (-38.1464, -10.9601) projected
  arc A46 (-38.3006, -14.9086) -> (-38.1464, -10.9601) centre (-40.4793, -12.8463) ccw projected
  arc A47 (35.5101, -49.1208) -> (36.1395, -40.0014) centre (-10.3402, -41.375) ccw projected
  arc A48 (31.8495, -51.5377) -> (35.5101, -49.1208) centre (32.552, -48.6211) ccw projected
  line L13 (31.8495, -51.5377) -> (29.9002, -51.0682) projected
  arc A49 (27.643, -47.6617) -> (29.9002, -51.0682) centre (30.6028, -48.1516) ccw projected
  arc A50 (27.643, -47.6617) -> (28.1492, -40.4742) centre (-10.3402, -41.375) ccw projected
  arc A51 (30.6814, -37.4406) -> (28.1492, -40.4742) centre (31.1484, -40.404) ccw projected
  line L14 (30.6814, -37.4406) -> (32.6737, -37.1266) projected
  arc A52 (36.1395, -40.0014) -> (32.6737, -37.1266) centre (33.1408, -40.09) ccw projected
  arc A53 (-27.4437, -78.8679) -> (-28.8048, -75.1583) centre (-30.2436, -77.7907) ccw projected
  line L15 (-27.4437, -78.8679) -> (-28.1679, -80.7504) projected
  arc A54 (-32.3905, -82.3144) -> (-28.1679, -80.7504) centre (-30.9679, -79.6732) ccw projected
  arc A55 (-39.9735, -77.2096) -> (-32.3905, -82.3144) centre (-10.3402, -41.375) ccw projected
  arc A56 (-40.2362, -72.831) -> (-39.9735, -77.2096) centre (-38.0617, -74.8977) ccw projected
  line L16 (-40.2362, -72.831) -> (-38.855, -71.3777) projected
  arc A57 (-34.7763, -71.1261) -> (-38.855, -71.3777) centre (-36.6804, -73.4444) ccw projected
  arc A58 (-34.7763, -71.1261) -> (-28.8048, -75.1583) centre (-10.3402, -41.375) ccw projected
  arc A59 (6.7633, -3.8821) -> (8.1244, -7.5917) centre (9.5632, -4.9593) ccw projected
  line L17 (6.7633, -3.8821) -> (9.1152, 2.2311) projected
  arc A60 (13.3061, 3.8119) -> (9.1152, 2.2311) centre (11.9151, 1.1538) ccw projected
  arc A61 (22.4148, -2.2839) -> (13.3061, 3.8119) centre (-10.3402, -41.375) ccw projected
  arc A62 (22.6626, -6.6501) -> (22.4148, -2.2839) centre (20.488, -4.5834) ccw projected
  line L18 (22.6626, -6.6501) -> (18.1745, -11.3723) projected
  arc A63 (14.0959, -11.6239) -> (18.1745, -11.3723) centre (16, -9.3056) ccw projected
  arc A64 (14.0959, -11.6239) -> (8.1244, -7.5917) centre (-10.3402, -41.375) ccw projected
  line L19 (21.5841, -76.8832) -> (17.466, -71.7899) projected
  arc A65 (17.6201, -67.8414) -> (17.466, -71.7899) centre (19.7989, -69.9037) ccw projected
  arc A66 (17.6201, -67.8414) -> (22.062, -62.168) centre (-10.3402, -41.375) ccw projected
  arc A67 (26.0203, -61.1529) -> (22.062, -62.168) centre (24.5868, -63.7882) ccw projected
  line L20 (26.0203, -61.1529) -> (31.7432, -64.2658) projected
  arc A68 (32.8503, -68.4965) -> (31.7432, -64.2658) centre (30.3097, -66.9011) ccw projected
  arc A69 (26.0581, -77.0984) -> (32.8503, -68.4965) centre (-10.3402, -41.375) ccw projected
  arc A70 (21.5841, -76.8832) -> (26.0581, -77.0984) centre (23.917, -74.997) ccw projected
  line L21 (-57.0534, -51.2682) -> (-50.5834, -50.2485) projected
  arc A71 (-47.2409, -52.3562) -> (-50.5834, -50.2485) centre (-50.1163, -53.2119) ccw projected
  arc A72 (-47.2409, -52.3562) -> (-44.5486, -59.0396) centre (-10.3402, -41.375) ccw projected
  arc A73 (-45.6486, -62.9752) -> (-44.5486, -59.0396) centre (-47.2142, -60.4161) ccw projected
  line L22 (-45.6486, -62.9752) -> (-51.2059, -66.3749) projected
  arc A74 (-55.4234, -65.2184) -> (-51.2059, -66.3749) centre (-52.7715, -63.8158) ccw projected
  arc A75 (-59.4768, -55.0352) -> (-55.4234, -65.2184) centre (-10.3402, -41.375) ccw projected
  arc A76 (-57.0534, -51.2682) -> (-59.4768, -55.0352) centre (-56.5864, -54.2316) ccw projected
  arc A77 (-34.2583, -7.8165) -> (-30.3651, -8.4926) centre (-31.9255, -5.9303) ccw projected
  line L23 (-34.2583, -7.8165) -> (-38.3765, -2.7231) projected
  arc A78 (-37.6501, 1.6967) -> (-38.3765, -2.7231) centre (-36.0436, -0.8369) ccw projected
  arc A79 (-27.8166, 6.5372) -> (-37.6501, 1.6967) centre (-10.3402, -41.375) ccw projected
  arc A80 (-23.9115, 4.5687) -> (-27.8166, 6.5372) centre (-26.7886, 3.7188) ccw projected
  line L24 (-23.9115, 4.5687) -> (-22.0659, -1.6792) projected
  arc A81 (-23.8874, -5.3372) -> (-22.0659, -1.6792) centre (-24.943, -2.529) ccw projected
  arc A82 (-23.8874, -5.3372) -> (-30.3651, -8.4926) centre (-10.3402, -41.375) ccw projected
  line L25 (31.8953, -32.1875) -> (29.9029, -32.5015) projected
  arc A83 (26.5605, -30.3938) -> (29.9029, -32.5015) centre (29.4359, -29.5381) ccw projected
  arc A84 (26.5605, -30.3938) -> (23.8681, -23.7104) centre (-10.3402, -41.375) ccw projected
  arc A85 (24.9682, -19.7748) -> (23.8681, -23.7104) centre (26.5337, -22.3339) ccw projected
  line L26 (24.9682, -19.7748) -> (26.6785, -18.7285) projected
  arc A86 (30.905, -19.9023) -> (26.6785, -18.7285) centre (28.2441, -21.2876) ccw projected
  arc A87 (34.3088, -28.3861) -> (30.905, -19.9023) centre (-10.3402, -41.375) ccw projected
  arc A88 (31.8953, -32.1875) -> (34.3088, -28.3861) centre (31.4283, -29.2241) ccw projected
  circle A89 centre (-81.1726, -30.4864) radius 2.1 projected
  circle A90 centre (-65.5868, -14.9006) radius 2.1 projected
  circle A91 centre (-101.657, -38.6244) radius 2.1 projected
  circle A92 centre (-57.4488, 5.5838) radius 2.1 projected
  circle A93 centre (-78.9982, -45.7929) radius 8 projected
  line L27 (-61.2813, 11.0455) -> (-50.1121, 17.3163) projected
  arc A94 (-102.4384, -34.1927) -> (-61.2813, 11.0455) centre (-111.1209, 15.0476) ccw projected
  line L28 (-102.4384, -34.1927) -> (-110.7406, -35.6566) projected
  line L29 (-110.7406, -35.6566) -> (-106.6609, -58.794) projected
  line L30 (-106.6609, -58.794) -> (-103.0049, -58.1494) projected
  arc A95 (-103.0049, -58.1494) -> (-82.3987, -72.578) centre (-78.9982, -45.7929) ccw projected
  line L31 (-82.3987, -72.578) -> (-81.7541, -76.234) projected
  line L32 (-81.7541, -76.234) -> (-73.8756, -74.8448) projected
  line L33 (-73.8756, -74.8448) -> (-28.2963, -90.7089) projected
  line L34 (-28.2963, -90.7089) -> (-30.7152, -97.3549) projected
  line L35 (-30.7152, -97.3549) -> (-15.0425, -100.6253) projected
  arc A96 (-15.0425, -100.6253) -> (-9.8606, -100.8097) centre (-10.3402, -41.375) ccw projected
  line L36 (-9.8606, -100.8097) -> (-9.8684, -99.8389) projected
  arc A97 (-7.953, -97.8245) -> (-9.8684, -99.8389) centre (-7.8685, -99.8228) ccw projected
  arc A98 (-7.953, -97.8245) -> (0.7138, -96.7831) centre (-10.3402, -41.375) ccw projected
  arc A99 (3.052, -98.2863) -> (0.7138, -96.7831) centre (1.1051, -98.7445) ccw projected
  line L37 (3.052, -98.2863) -> (3.358, -99.5868) projected
  arc A100 (3.358, -99.5868) -> (9.3677, -97.836) centre (-10.3402, -41.375) ccw projected
  line L38 (9.3677, -97.836) -> (20.2434, -92.7646) projected
  arc A101 (20.2434, -92.7646) -> (25.4476, -89.2862) centre (-10.3402, -41.375) ccw projected
  line L39 (25.4476, -89.2862) -> (24.6481, -88.2159) projected
  arc A102 (24.9994, -85.4585) -> (24.6481, -88.2159) centre (26.2504, -87.019) ccw projected
  arc A103 (24.9994, -85.4585) -> (31.3681, -79.4888) centre (-10.3402, -41.375) ccw projected
  arc A104 (34.1424, -79.3163) -> (31.3681, -79.4888) centre (32.8445, -80.838) ccw projected
  line L40 (34.1424, -79.3163) -> (34.8811, -79.9463) projected
  arc A105 (34.8811, -79.9463) -> (38.0707, -75.8583) centre (-10.3402, -41.375) ccw projected
  line L41 (38.0707, -75.8583) -> (45.6397, -61.75) projected
  line L42 (45.6397, -61.75) -> (38.9936, -59.3311) projected
  arc A106 (38.9936, -59.3311) -> (35.1261, -15.125) centre (-10.3402, -41.375) ccw projected
  line L43 (35.1261, -15.125) -> (41.2511, -11.5887) projected
  line L44 (41.2511, -11.5887) -> (31.3473, 0.9908) projected
  arc A107 (31.3473, 0.9908) -> (27.4962, 4.4629) centre (-10.3402, -41.375) ccw projected
  line L45 (27.4962, 4.4629) -> (26.8782, 3.7142) projected
  arc A108 (24.1161, 3.4024) -> (26.8782, 3.7142) centre (25.3358, 4.9874) ccw projected
  arc A109 (24.1161, 3.4024) -> (16.8075, 8.1755) centre (-10.3402, -41.375) ccw projected
  arc A110 (15.9827, 10.8299) -> (16.8075, 8.1755) centre (17.7685, 9.9295) ccw projected
  line L46 (15.9827, 10.8299) -> (16.5842, 12.0228) projected
  arc A111 (16.5842, 12.0228) -> (10.8551, 14.5447) centre (-10.3402, -41.375) ccw projected
  line L47 (10.8551, 14.5447) -> (-0.736, 17.6505) projected
  arc A112 (-0.736, 17.6505) -> (-6.9585, 18.3311) centre (-10.3402, -41.375) ccw projected
  line L48 (-6.9585, 18.3311) -> (-7.034, 16.9972) projected
  arc A113 (-9.0756, 15.1108) -> (-7.034, 16.9972) centre (-9.0308, 17.1103) ccw projected
  arc A114 (-9.0756, 15.1108) -> (-17.7916, 14.6315) centre (-10.3402, -41.375) ccw projected
  arc A115 (-20.0277, 16.2826) -> (-17.7916, 14.6315) centre (-18.0553, 16.614) ccw projected
  line L49 (-20.0277, 16.2826) -> (-20.1886, 17.24) projected
  arc A116 (-20.1886, 17.24) -> (-25.2597, 16.1586) centre (-10.3402, -41.375) ccw projected
  line L50 (-25.2597, 16.1586) -> (-40.1265, 10.2163) projected
  line L51 (-40.1265, 10.2163) -> (-50.1121, 17.3163) projected
  circle A117 centre (-103.9086, -54.247) radius 1.5 projected
  circle A118 centre (-13.7974, -97.2048) radius 1.5 projected
  circle A119 centre (20.8436, -88.2521) radius 1.5 projected
  circle A120 centre (28.1949, -0.8291) radius 1.5 projected
  circle A121 centre (-4.0964, 14.5795) radius 1.5 projected
  circle A122 centre (-23.4396, 13.0063) radius 1.5 projected
  circle A123 centre (12.2297, 10.2049) radius 1.5 projected
  circle A124 centre (34.6501, -74.6133) radius 1.5 projected
  circle A125 centre (5.5251, -95.3952) radius 1.5 projected
  circle A126 centre (-78.4226, -72.0925) radius 1.5 projected
  circle A127 centre (-10.3402, -41.375) radius 32.5 projected
  line L52 (24.5868, -63.7882) -> (30.6028, -48.1516)
  line L53 (-10.3402, -41.375) -> (27.5948, -55.9699)
  circle A128 centre (-10.3402, -41.375) radius 32.5 projected
  circle A129 centre (19.9923, -53.045) radius 2.5
  point P0 (0, 0)
  dimension "d79" = 5
  constraints: 4 end point, 1 centre point, 1 midpoint, 1 point on line, 2 other
  measures "d79" diameter of A129
extrude "Extrusion13" cut sketch "Sketch15" against normal blind 5 contours A129 L53 A127 | A127 L53 A129 | A129 L53 A127 | A127 L53 A129
pattern_circular "Circular Pattern1" count 6 over 360 about axis through (-10.3402, -41.375, 5) along (0, 0, -1) of "Extrusion13"
fillet "Fillet6" radius 2 7 edges at (-28.2963, -90.7089, 2.5) (38.9936, -59.3311, 2.5) (35.1261, -15.125, 2.5) (-40.1265, 10.2163, 2.5) (-82.3987, -72.578, 2.5) (-103.0049, -58.1494, 2.5) (-73.8756, -74.8448, 2.5)
body "Solid1"
